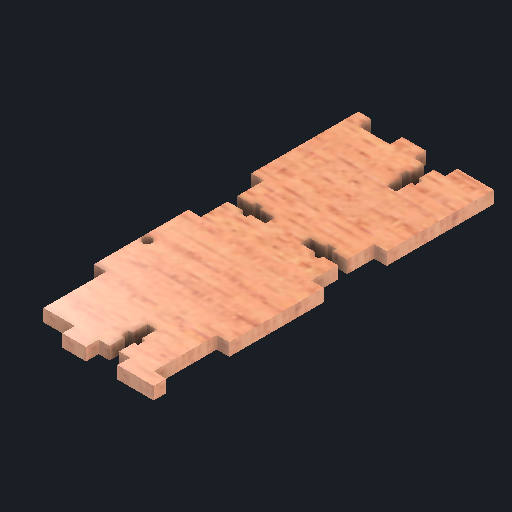
# Autodesk Inventor part: FloorButtonHolder_Bottom_V1
Saved by Autodesk Inventor 2024.1 (Build 281209000, 209)
## iProperties
Created: 2023-05-20
Part Number: FloorButtonHolder_Bottom_V1
Material: MDF Medium Density Fiberboard
Document SubType Name: Modeling
Designer: jaege
Density: 0.8 g/cm^3
Appearance: Red Oak - Natural Low Gloss
Author: jaege
Autodesk Inventor part; units mm, degrees
ref_plane "YZ Plane" through (0, 0, 0) normal (1, 0, 0) x (0, 1, 0)
ref_plane "XZ Plane" through (0, 0, 0) normal (0, 1, 0) x (-1, 0, 0)
ref_plane "XY Plane" through (0, 0, 0) normal (0, 0, 1) x (1, 0, 0)
sketch "Sketch1" plane through (0, 0, 0) normal (0, 1, 0) x (-1, 0, 0)
  line L0 (-17.5, 50) -> (17.5, 50)
  line L1 (17.5, 50) -> (17.5, -50)
  line L2 (17.5, -50) -> (-17.5, -50)
  line L3 (-17.5, -50) -> (-17.5, 50)
  line L4 (-17.5, 50) -> (17.5, -50) construction
  line L5 (17.5, 50) -> (-17.5, -50) construction
  line L6 (7.5, 50) -> (0, 50)
  line L7 (0, 50) -> (0, 54)
  line L8 (0, 54) -> (7.5, 54)
  line L9 (7.5, 54) -> (7.5, 50)
  line L10 (-10, 50) -> (-21.5, 50)
  line L11 (-21.5, 50) -> (-21.5, 54)
  line L12 (-21.5, 54) -> (-10, 54)
  line L13 (-10, 54) -> (-10, 50)
  line L14 (17.5, 30) -> (21.5, 30)
  line L15 (21.5, 30) -> (21.5, 0)
  line L16 (21.5, 0) -> (17.5, 0)
  line L17 (17.5, 0) -> (17.5, 30)
  line L18 (17.5, -20) -> (21.5, -20)
  line L19 (21.5, -20) -> (21.5, -54)
  line L20 (21.5, -54) -> (17.5, -54)
  line L21 (17.5, -54) -> (17.5, -20)
  line L22 (7.5, -50) -> (0, -50)
  line L23 (0, -50) -> (0, -54)
  line L24 (0, -54) -> (7.5, -54)
  line L25 (7.5, -54) -> (7.5, -50)
  line L26 (-10, -50) -> (-21.5, -50)
  line L27 (-21.5, -50) -> (-21.5, -54)
  line L28 (-21.5, -54) -> (-10, -54)
  line L29 (-10, -54) -> (-10, -50)
  line L30 (-17.5, 30) -> (-21.5, 30)
  line L31 (-21.5, 30) -> (-21.5, 0)
  line L32 (-21.5, 0) -> (-17.5, 0)
  line L33 (-17.5, 0) -> (-17.5, 30)
  line L34 (-17.5, -50) -> (-21.5, -50)
  line L35 (-21.5, -50) -> (-21.5, -20)
  line L36 (-21.5, -20) -> (-17.5, -20)
  line L37 (-17.5, -20) -> (-17.5, -50)
  point P0 (0, 0)
  point P1 (17.5, 0)
  point P2 (-17.5, 50)
  point P3 (-17.5, 0)
  point P4 (17.5, -50)
  point P5 (19.5, -54)
  dimension "d0" = 35
  dimension "d2" = 7.5
  dimension "d3" = 4
  dimension "d4" = 11.5
  dimension "d5" = 4
  dimension "d6" = 10
  dimension "d7" = 10
  dimension "d8" = 4
  dimension "d9" = 30
  dimension "d10" = 4
  dimension "d11" = 34
  dimension "d12" = 20
  dimension "d13" = 20
  dimension "d14" = 7.5
  dimension "d15" = 4
  dimension "d16" = 11.5
  dimension "d17" = 4
  dimension "d18" = 10
  dimension "d19" = 10
  dimension "d20" = 4
  dimension "d21" = 30
  dimension "d22" = 20
  dimension "d23" = 4
  dimension "d24" = 30
  dimension "d27" = 4
  constraints: 76 end point, 18 parallel, 9 horizontal, 9 perpendicular, 7 point on line, 3 midpoint
  measures "d0" distance of L1.end L2.end
  measures "d2" distance of L7.end L8.end
  measures "d3" distance of L6.end L7.end
  measures "d4" distance of L11.end L12.end
  measures "d5" distance of L10.end L11.end
  measures "d6" distance between parallel lines of L9 L1
  measures "d7" distance between parallel lines of L13 L7
  measures "d8" distance of L15.end L16.end
  measures "d9" distance of L14.end L15.end
  measures "d10" distance of L19.end L20.end
  measures "d11" distance of L18.end L19.end
  measures "d12" distance between parallel lines of L16 L18
  measures "d13" distance between parallel lines of L0 L14
  measures "d14" distance of L24.end L23.end
  measures "d15" distance of L23.end L22.end
  measures "d16" distance of L28.end L27.end
  measures "d17" distance of L27.end L26.end
  measures "d18" distance between parallel lines of L25 L21
  measures "d19" distance between parallel lines of L29 L23
  measures "d20" distance of L32.end L31.end
  measures "d21" distance of L31.end L30.end
  measures "d22" distance between parallel lines of L10 L30
  measures "d23" distance of L35.end L36.end
  measures "d24" distance of L34.end L35.end
  measures "d27" distance from line of L2 point (19.5, -54)
extrude "Extrusion1" add sketch "Sketch1" along normal blind 4
sketch "Sketch2" plane through (0, 0, 0) normal (0, -1, 0) x (1, 0, 0)
  line L0 (6.5, 45.2) -> (6.5, 50) projected
  line L1 (6.5, 50) -> (10, 50) construction
  line L2 (10, 50) -> (10, 54) construction
  line L3 (10, 54) -> (21.5, 54) construction
  line L4 (21.5, 54) -> (21.5, 50) construction
  line L5 (21.5, 50) -> (17.5, 50) construction
  line L6 (17.5, 50) -> (17.5, 30) construction
  line L7 (17.5, 30) -> (21.5, 30) construction
  line L8 (21.5, 30) -> (21.5, 0) construction
  line L9 (21.5, 0) -> (17.5, 0) construction
  line L10 (17.5, 0) -> (17.5, -8.5) construction
  line L11 (17.5, -8.5) -> (12.7, -8.5) projected
  line L12 (12.7, -8.5) -> (12.7, -7.3) projected
  line L13 (12.7, -7.3) -> (10.3, -7.3) projected
  line L14 (10.3, -7.3) -> (10.3, -8.5) projected
  line L15 (10.3, -8.5) -> (5.5, -8.5) projected
  line L16 (5.5, -8.5) -> (5.5, -11.5) projected
  line L17 (5.5, -11.5) -> (10.3, -11.5) projected
  line L18 (10.3, -11.5) -> (10.3, -12.7) projected
  line L19 (10.3, -12.7) -> (12.7, -12.7) projected
  line L20 (12.7, -12.7) -> (12.7, -11.5) projected
  line L21 (12.7, -11.5) -> (17.5, -11.5) projected
  line L22 (17.5, -11.5) -> (17.5, -20) construction
  line L23 (17.5, -20) -> (21.5, -20) construction
  line L24 (21.5, -20) -> (21.5, -54) construction
  line L25 (21.5, -54) -> (10, -54) construction
  line L26 (10, -54) -> (10, -50) construction
  line L27 (10, -50) -> (6.5, -50) construction
  line L28 (6.5, -50) -> (6.5, -45.2) projected
  line L29 (6.5, -45.2) -> (7.7, -45.2) projected
  line L30 (7.7, -45.2) -> (7.7, -42.8) projected
  line L31 (7.7, -42.8) -> (6.5, -42.8) projected
  line L32 (6.5, -42.8) -> (6.5, -38) projected
  line L33 (6.5, -38) -> (3.5, -38) projected
  line L34 (3.5, -38) -> (3.5, -42.8) projected
  line L35 (3.5, -42.8) -> (2.3, -42.8) projected
  line L36 (2.3, -42.8) -> (2.3, -45.2) projected
  line L37 (2.3, -45.2) -> (3.5, -45.2) projected
  line L38 (3.5, -45.2) -> (3.5, -50) projected
  line L39 (3.5, -50) -> (0, -50) projected
  line L40 (0, -50) -> (0, -54) construction
  line L41 (0, -54) -> (-7.5, -54) construction
  line L42 (-7.5, -54) -> (-7.5, -50) construction
  line L43 (-7.5, -50) -> (-17.5, -50) construction
  line L44 (-17.5, -50) -> (-17.5, -54) construction
  line L45 (-17.5, -54) -> (-21.5, -54) construction
  line L46 (-21.5, -54) -> (-21.5, -20) construction
  line L47 (-21.5, -20) -> (-17.5, -20) construction
  line L48 (-17.5, -20) -> (-17.5, -11.5) construction
  line L49 (-17.5, -11.5) -> (-12.7, -11.5) projected
  line L50 (-12.7, -11.5) -> (-12.7, -12.7) projected
  line L51 (-12.7, -12.7) -> (-10.3, -12.7) projected
  line L52 (-10.3, -12.7) -> (-10.3, -11.5) projected
  line L53 (-10.3, -11.5) -> (-5.5, -11.5) projected
  line L54 (-5.5, -11.5) -> (-5.5, -8.5) projected
  line L55 (-5.5, -8.5) -> (-10.3, -8.5) projected
  line L56 (-10.3, -8.5) -> (-10.3, -7.3) projected
  line L57 (-10.3, -7.3) -> (-12.7, -7.3) projected
  line L58 (-12.7, -7.3) -> (-12.7, -8.5) projected
  line L59 (-12.7, -8.5) -> (-17.5, -8.5) projected
  line L60 (-17.5, -8.5) -> (-17.5, 0) construction
  line L61 (-17.5, 0) -> (-21.5, 0) construction
  line L62 (-21.5, 0) -> (-21.5, 30) construction
  line L63 (-21.5, 30) -> (-17.5, 30) construction
  line L64 (-17.5, 30) -> (-17.5, 50) construction
  line L65 (-17.5, 50) -> (-7.5, 50) construction
  line L66 (-7.5, 50) -> (-7.5, 54) construction
  line L67 (-7.5, 54) -> (0, 54) construction
  line L68 (0, 54) -> (0, 50) construction
  line L69 (0, 50) -> (3.5, 50) projected
  line L70 (3.5, 50) -> (3.5, 45.2) projected
  line L71 (3.5, 45.2) -> (2.3, 45.2) projected
  line L72 (2.3, 45.2) -> (2.3, 42.8) projected
  line L73 (2.3, 42.8) -> (3.5, 42.8) projected
  line L74 (3.5, 42.8) -> (3.5, 38) projected
  line L75 (3.5, 38) -> (6.5, 38) projected
  line L76 (6.5, 38) -> (6.5, 42.8) projected
  line L77 (6.5, 42.8) -> (7.7, 42.8) projected
  line L78 (7.7, 42.8) -> (7.7, 45.2) projected
  line L79 (7.7, 45.2) -> (6.5, 45.2) projected
  circle A0 centre (-19.5, 15) radius 1.5 projected
  line L80 (3.5, 50) -> (6.5, 50)
  line L81 (0, 50) -> (10, 50) projected
  line L82 (-17.5, -8.5) -> (-17.5, -11.5)
  line L83 (3.5, -50) -> (6.5, -50)
  line L84 (10, -50) -> (0, -50) projected
  line L85 (17.5, -11.5) -> (17.5, -8.5)
  point P0 (0, 0)
  constraints: 8 end point, 3 collinear, 1 perpendicular
extrude "Extrusion2" cut sketch "Sketch2" against normal up to next
body "Solid1"
